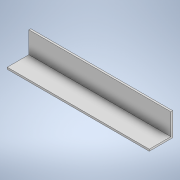
# Autodesk Inventor part: AluminiumAngle
Saved by Autodesk Inventor 2020 (Build 240168000, 168)
## iProperties
Created: 2020-03-05
Part Number: AluminiumAngle
Material: Generic
Document SubType Name: Modeling
Designer: 19673418
Density: 1 g/cm^3
Appearance: Default
Author: 19673418
Autodesk Inventor part; units mm, degrees
ref_plane "YZ Plane" through (0, 0, 0) normal (1, 0, 0) x (0, 1, 0)
ref_plane "XZ Plane" through (0, 0, 0) normal (0, 1, 0) x (-1, 0, 0)
ref_plane "XY Plane" through (0, 0, 0) normal (0, 0, 1) x (1, 0, 0)
sketch "Sketch1" plane through (0, 0, 0) normal (0, 0, 1) x (1, 0, 0)
  line L0 (0, 0) -> (230, 0)
  line L1 (230, 0) -> (230, 38)
  line L2 (230, 38) -> (0, 38)
  line L3 (0, 38) -> (0, 0)
  dimension "d0" = 230
  dimension "d1" = 38
  constraints: 8 end point, 2 parallel, 1 horizontal, 1 perpendicular
  measures "d0" distance of L2.end L1.end
  measures "d1" distance of L1.end L0.end
extrude "Extrusion1" add sketch "Sketch1" against normal blind 3
sketch "Sketch2" plane through (0, 0, 0) normal (0, 0, 1) x (1, 0, 0)
  line L0 (0, 0) -> (0, 38) projected
  line L1 (0, 0) -> (230, 0)
  line L2 (230, 0) -> (230, 3)
  line L3 (230, 3) -> (0, 3)
  line L4 (0, 3) -> (0, 0)
  dimension "d4" = 230
  dimension "d5" = 3
  constraints: 8 end point, 2 parallel, 1 horizontal, 1 perpendicular
  measures "d4" distance of L3.end L2.end
  measures "d5" distance of L2.end L1.end
extrude "Extrusion2" add sketch "Sketch2" along normal blind 35
body "Solid1"
